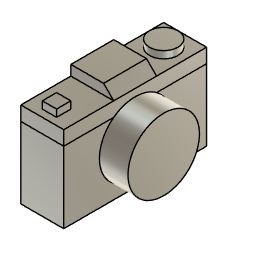
3rd (Autodesk Fusion 360 design; units mm, degrees)
part number: 2025-09-11-11-23-15-718
Autodesk Fusion 360 part; units mm, degrees
note: some values were not read from the file. Set by a fixed rule: which sketch regions a step uses.
sketch "Sketch1" plane through (0, 0, 0) normal (1, 0, 0) x (0, 1, 0)
  line L0 (50, -25) -> (-50, -25)
  line L1 (-50, -25) -> (-50, 25)
  line L2 (-50, 25) -> (50, 25)
  line L3 (50, 25) -> (50, -25)
  line L4 (50, -25) -> (-50, 25) construction
  line L5 (-50, -25) -> (50, 25) construction
  dimension "d1" = 100
  dimension "d2" = 50
  constraint horizontal L0
  constraint perpendicular L0 L1
  constraint parallel L0 L2
  constraint parallel L1 L3
  constraint coincident L4 origin
  constraint coincident L5 origin
  measures "d1" distance of L1.end L2.end
  measures "d2" distance of L0.end L1.end
extrude "Extrude1" add sketch "Sketch1" along normal blind 30 makes body 1
sketch "Sketch2" plane through (0, 0, 25) normal (0, 0, 1) x (-1, 0, 0)
  line L0 (0, -50) -> (0, 50)
  line L1 (0, 50) -> (-30, 50)
  line L2 (-30, 50) -> (-30, -50)
  line L3 (-30, -50) -> (0, -50)
  line L4 (0, 50) -> (-15, 50)
  line L5 (-15, 50) -> (-15, 0)
  line L6 (-30, 50) -> (0, 50)
  line L7 (0, 50) -> (0, -50)
  line L8 (0, -50) -> (-30, -50)
  line L9 (-30, -50) -> (-30, 50)
  line L10 (-30, 50) -> (0, -50) construction
  line L11 (0, 50) -> (-30, -50) construction
  point P0 (-15, 0)
  constraint coincident L0.end L1.start
  constraint midpoint L1 L4.end
  constraint perpendicular L1 L5
  constraint horizontal L6
  constraint perpendicular L6 L7
  constraint parallel L6 L8
  constraint parallel L7 L9
  constraint coincident L10 P0
  constraint coincident L11 P0
  constraint coincident P0 L5.end
extrude "Extrude2" add sketch "Sketch2" along normal blind 10 separate body makes body 2
sketch "Sketch3" plane through (30, 0, 0) normal (1, 0, 0) x (0, 1, 0)
  line L0 (50, 25) -> (-50, 25)
  line L1 (-50, 25) -> (-50, -25)
  line L2 (-50, -25) -> (50, -25)
  line L3 (50, -25) -> (50, 25)
  line L4 (-50, 35) -> (-50, 5)
  line L5 (-50, 35) -> (0, 35)
  circle A0 centre (0, 5) radius 25
  dimension "d7" = 30
  dimension "d8" = 50
  constraint perpendicular L0 L4
  constraint perpendicular L4 L5
  measures "d7" distance of L4.start L4.end
  measures "d8" diameter of A0
extrude "Extrude3" add sketch "Sketch3" along normal blind 20 separate body contours L0 A0 | L0 A0 makes body 3
sketch "Sketch4" plane through (0, 0, 35) normal (0, 0, 1) x (-1, 0, 0)
  line L0 (-30, -50) -> (0, -50)
  line L1 (0, -50) -> (0, 50)
  line L2 (0, 50) -> (-30, 50)
  line L3 (-30, 50) -> (-30, -50)
  line L4 (0, 50) -> (-15, 50)
  line L5 (-15, 50) -> (-15, 40)
  line L6 (-10, 35) -> (-20, 35)
  line L7 (-20, 35) -> (-20, 45)
  line L8 (-20, 45) -> (-10, 45)
  line L9 (-10, 45) -> (-10, 35)
  point P0 (-15, 40)
  dimension "d11" = 10
  dimension "d12" = 10
  dimension "d13" = 10
  constraint coincident L1.end L2.start
  constraint midpoint L2 L4.end
  constraint perpendicular L2 L5
  constraint horizontal L6
  constraint perpendicular L6 L7
  constraint parallel L6 L8
  constraint parallel L7 L9
  constraint coincident P0 L5.end
  measures "d11" distance of L4.end P0
  measures "d12" distance of L7.end L8.end
  measures "d13" distance of L6.end L7.end
extrude "Extrude4" add sketch "Sketch4" along normal blind 5 separate body contours L6 L7 L8 L9 makes body 4
sketch "Sketch5" plane through (0, 0, 35) normal (0, 0, 1) x (-1, 0, 0)
  line L0 (-30, -50) -> (0, -50)
  line L1 (0, -50) -> (0, 50)
  line L2 (0, 50) -> (-30, 50)
  line L3 (-30, 50) -> (-30, -50)
  line L4 (-30, -50) -> (-15, -50)
  line L5 (-15, -50) -> (-15, -35)
  circle A0 centre (-15, -35) radius 10
  dimension "d16" = 15
  dimension "d17" = 20
  constraint coincident L0.start L3.end
  constraint midpoint L0 L4.end
  constraint perpendicular L4 L5
  constraint coincident L5.end A0.centre
  measures "d16" distance of L4.end L5.end
  measures "d17" diameter of A0
extrude "Extrude5" add sketch "Sketch5" along normal blind 5 contours A0 bodies 2
ref_plane "WorkPlane1" through (15, 0, 0) normal (0, 1, 0) x (0, 0, 1)
sketch "Sketch6" plane through (0, 0, 0) normal (0, 1, 0) x (1, 0, 0)
ref_plane "WorkPlane2" through (15, 0, 0) normal (0, 1, 0) x (0, 0, 1)
sketch "Sketch7" plane through (0, 0, 0) normal (0, 1, 0) x (1, 0, 0)
  line L0 (30, -35) -> (22.9289, -42.0711)
  line L1 (30, -35) -> (40, -35) construction
  line L2 (22.9289, -42.0711) -> (0, -42.0711)
  line L3 (0, -42.0711) -> (0, -35)
  line L4 (0, -35) -> (30, -35)
  dimension "d20" = 135
  dimension "d21" = 10
  constraint horizontal L1
  constraint horizontal L2
  constraint perpendicular L2 L3
  constraint perpendicular L3 L4
  measures "d20" angle of L0 L1
  measures "d21" distance of L0.start L0.end
extrude "Extrude6" add sketch "Sketch7" along normal blind 15 and the other way blind 15 bodies 2
